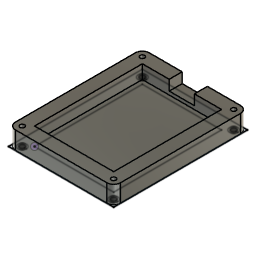
Zohair Keyboard v2 (Autodesk Fusion 360 design; units mm, degrees)
Autodesk Fusion 360 part; units mm, degrees
sketch "Sketch1" plane through (0, 0, 0) normal (0, 0, 1) x (1, 0, 0)
  line L0 (0, 0) -> (58.025, 0)
  line L1 (58.025, 0) -> (58.025, 79.025)
  line L2 (58.025, 79.025) -> (0, 79.025)
  line L3 (0, 79.025) -> (0, 0)
  line L4 (-9.5, -9.5) -> (67.525, -9.5)
  line L5 (67.525, -9.5) -> (67.525, 88.525)
  line L6 (67.525, 88.525) -> (-9.5, 88.525)
  line L7 (-9.5, 88.525) -> (-9.5, -9.5)
  circle A0 centre (-4.5, -4.5) radius 1.7
  circle A1 centre (-4.5, 83.525) radius 1.7
  circle A2 centre (62.525, 83.525) radius 1.7
  circle A3 centre (-4.5, -4.5) radius 3
  circle A4 centre (62.525, -4.5) radius 1.7
  circle A5 centre (62.525, -4.5) radius 3
  circle A6 centre (-4.5, 83.525) radius 3
  circle A7 centre (62.525, 83.525) radius 3
  dimension "d1" = 58.025
  dimension "d2" = 79.025
  dimension "d3" = 77.025
  dimension "d4" = 98.025
  dimension "d5" = 9.5
  dimension "d6" = 9.5
  dimension "d11" = 3.4
  dimension "d12" = 5
  dimension "d13" = 5
  dimension "d14" = 3.4
  dimension "d15" = 5
  dimension "d16" = 5
  dimension "d17" = 3.4
  dimension "d18" = 5
  dimension "d19" = 5
  dimension "d20" = 6
  dimension "d21" = 3.4
  dimension "d22" = 5
  dimension "d23" = 5
  dimension "d24" = 6
  dimension "d25" = 6
  dimension "d26" = 6
  constraint horizontal L0
  constraint vertical L1
  constraint horizontal L2
  constraint vertical L3
  constraint coincident L0.start L3.end
  constraint horizontal L4
  constraint vertical L5
  constraint horizontal L6
  constraint vertical L7
  constraint concentric A0 A3
  constraint concentric A4 A5
  constraint concentric A1 A6
  constraint concentric A2 A7
  measures "d1" distance of L0.start L0.end
  measures "d2" distance of L0.start L2.end
  measures "d3" distance of L4.start L4.end
  measures "d4" distance of L4.start L6.end
  measures "d5" distance of L2 L6
  measures "d6" distance of L3 L7
  measures "d11" diameter of A0
  measures "d12" distance of L7 A0.centre
  measures "d13" distance of L4 A0.centre
  measures "d14" diameter of A1
  measures "d15" distance of L6 A1.centre
  measures "d16" distance of L7 A1.centre
  measures "d17" diameter of A2
  measures "d18" distance of L6 A2.centre
  measures "d19" distance of L5 A2.centre
  measures "d20" diameter of A3
  measures "d21" diameter of A4
  measures "d22" distance of L4 A4.centre
  measures "d23" distance of L5 A4.centre
  measures "d24" diameter of A5
  measures "d25" diameter of A6
  measures "d26" diameter of A7
extrude "Extrude1" add sketch "Sketch1" along normal blind 9.9 from surface at 3.1 contours A3 | A5 | A6 | A7 makes body 1 at (59.7606, 82.3597, 9.7) makes body 2 at (-1.5037, -4.6495, 9.7) makes body 3 at (-7.0599, 81.9607, 9.7) makes body 4 at (65.5213, -4.6495, 9.7)
extrude "Extrude2" add sketch "Sketch1" along normal blind 13 contours L4 L5 L6 L7 bodies 1 2 3 4
extrude "Extrude3" add sketch "Sketch1" along normal blind 3 contours L0 L1 L2 L3 bodies 1
sketch "Sketch3" plane through (0, 0, 13) normal (0, 0, 1) x (-1, 0, 0)
  circle A0 centre (-62.525, -83.525) radius 1.7
  circle A1 centre (-62.525, 4.5) radius 1.7
  line L0 (0, 0) -> (0, -79.025)
  line L1 (0, -79.025) -> (-58.025, -79.025)
  line L2 (-58.025, -79.025) -> (-58.025, 0)
  line L3 (-58.025, 0) -> (0, 0)
  line L4 (9.5, -88.525) -> (9.5, 9.5)
  line L5 (9.5, 9.5) -> (-67.525, 9.5)
  line L6 (-67.525, 9.5) -> (-67.525, -88.525)
  line L7 (-67.525, -88.525) -> (9.5, -88.525)
  circle A2 centre (4.5, 4.5) radius 1.7
  circle A3 centre (4.5, -83.525) radius 1.7
  line L8 (-19.7, -88.525) -> (-38.2, -88.525)
  line L9 (-38.2, -88.525) -> (-38.2, -79.025)
  line L10 (-38.2, -79.025) -> (-19.7, -79.025)
  line L11 (-19.7, -79.025) -> (-19.7, -88.525)
  line L12 (9.5, -88.525) -> (9.5, 9.5)
  dimension "d36" = 18.5
  dimension "d37" = 29.2
  constraint horizontal L8
  constraint vertical L9
  constraint horizontal L10
  constraint vertical L11
  constraint coincident L7 L8.start
  measures "d36" distance of L8.start L8.end
  measures "d37" distance of L11 L12
extrude "Extrude4" cut sketch "Sketch3" against normal blind 7.5 contours L1 L7 L8 L9 L10 L11 bodies 1
fillet "Fillet1" radius 5 1 edges at (67.525, -9.5, 6.5) on bodies 1
fillet "Fillet2" radius 5 3 edges at (-9.5, -9.5, 6.5) (67.525, 88.525, 6.5) (-9.5, 88.525, 6.5) on bodies 1
